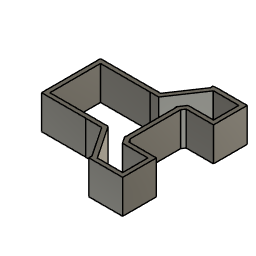
Duplex Sample Pad 1.5ScaleUp (Autodesk Fusion 360 design; units mm, degrees)
Autodesk Fusion 360 part; units mm, degrees
note: some values were not read from the file. Set by a fixed rule: which sketch regions a step uses.
sketch "Sketch1" plane through (0, 0, 0) normal (0, 0, 1) x (1, 0, 0)
  line L0 (5.0374, 3.1227) -> (6.2836, 3.1227)
  line L1 (6.2836, 3.1227) -> (6.2836, 5.3716)
  line L2 (6.2836, 5.3716) -> (4.024, 5.3716)
  line L3 (4.024, 5.3716) -> (4.024, 5.3478)
  line L4 (4.024, 5.3478) -> (2.0793, 2.4559)
  line L5 (2.0793, 2.4559) -> (1.3173, 2.4559)
  line L6 (1.3173, 2.4559) -> (1.3173, 2.4506)
  line L7 (1.3173, 2.4506) -> (-3.0986, 2.4506)
  line L8 (-3.0986, 2.4506) -> (-3.0986, -2.0499)
  line L9 (-3.0986, -2.0499) -> (0.9892, -2.0499)
  line L10 (0.9892, -2.0499) -> (0.9892, -2.0552)
  line L11 (0.9892, -2.0552) -> (2.0846, -2.0552)
  line L12 (2.0846, -2.0552) -> (4.0293, -4.9471)
  line L13 (4.0293, -4.9471) -> (4.0293, -4.9709)
  line L14 (4.0293, -4.9709) -> (6.2889, -4.9709)
  line L15 (6.2889, -4.9709) -> (6.2889, -2.722)
  line L16 (6.2889, -2.722) -> (5.0427, -2.722)
  line L17 (5.0427, -2.722) -> (4.0293, -2.722)
  line L18 (4.0293, -2.722) -> (3.5822, -2.0579)
  line L19 (3.5822, -2.0579) -> (3.6457, -2.0579)
  line L20 (3.6457, -2.0579) -> (3.6457, -2.0526)
  line L21 (3.6457, -2.0526) -> (3.6536, -2.0526)
  line L22 (3.6536, -2.0526) -> (3.6536, 2.448)
  line L23 (3.6536, 2.448) -> (3.6457, 2.448)
  line L24 (3.6457, 2.448) -> (3.6457, 2.4533)
  line L25 (3.6457, 2.4533) -> (3.5822, 2.4533)
  line L26 (3.5822, 2.4533) -> (4.0293, 3.1174)
  line L27 (4.0293, 3.1174) -> (5.0427, 3.1174)
  line L28 (5.0427, 3.1174) -> (5.0374, 3.1227)
  line L29 (4.2251, 2.7496) -> (6.6593, 2.7496)
  line L30 (6.6593, 2.7496) -> (6.6593, 5.75)
  line L31 (6.6593, 5.75) -> (4.024, 5.75)
  line L32 (4.024, 5.75) -> (3.6483, 5.7262)
  line L33 (3.6483, 5.7262) -> (3.6483, 5.4642)
  line L34 (3.6483, 5.4642) -> (1.8782, 2.8343)
  line L35 (1.8782, 2.8343) -> (1.3147, 2.8343)
  line L36 (1.3147, 2.8343) -> (0.9813, 2.829)
  line L37 (0.9813, 2.829) -> (-3.4743, 2.829)
  line L38 (-3.4743, 2.829) -> (-3.4743, -2.4204)
  line L39 (-3.4743, -2.4204) -> (0.4574, -2.4204)
  line L40 (0.4574, -2.4204) -> (0.4574, -2.4256)
  line L41 (0.4574, -2.4256) -> (1.8809, -2.4256)
  line L42 (1.8809, -2.4256) -> (3.651, -5.0556)
  line L43 (3.651, -5.0556) -> (3.651, -5.3387)
  line L44 (3.651, -5.3387) -> (6.6619, -5.3387)
  line L45 (6.6619, -5.3387) -> (6.6619, -2.3383)
  line L46 (6.6619, -2.3383) -> (4.2277, -2.3383)
  line L47 (4.2277, -2.3383) -> (4.0267, -2.0394)
  line L48 (4.0267, -2.0394) -> (4.0267, 2.4559)
  line L49 (4.0267, 2.4559) -> (4.2277, 2.7549)
  line L50 (4.2277, 2.7549) -> (4.2251, 2.7496)
  line L51 (3.6404, 2.4586) -> (3.6404, 2.4533)
  line L52 (3.6404, 2.4533) -> (3.6483, 2.4533)
  line L53 (3.6483, 2.4533) -> (3.6483, -2.0473)
  line L54 (3.6483, -2.0473) -> (3.6404, -2.0473)
  line L55 (3.6404, -2.0473) -> (3.6404, -2.0526)
  line L56 (3.6404, -2.0526) -> (3.5769, -2.0526)
  line L57 (3.5769, -2.0526) -> (4.024, -2.7167)
  line L58 (4.024, -2.7167) -> (5.0374, -2.7167)
  line L59 (5.0374, -2.7167) -> (6.2836, -2.7167)
  line L60 (6.2836, -2.7167) -> (6.2836, -4.9657)
  line L61 (6.2836, -4.9657) -> (4.024, -4.9657)
  line L62 (4.024, -4.9657) -> (4.024, -4.9418)
  line L63 (4.024, -4.9418) -> (2.0793, -2.0499)
  line L64 (2.0793, -2.0499) -> (0.9839, -2.0499)
  line L65 (0.9839, -2.0499) -> (0.9839, -2.0447)
  line L66 (0.9839, -2.0447) -> (-3.1039, -2.0447)
  line L67 (-3.1039, -2.0447) -> (-3.1039, 2.4559)
  line L68 (-3.1039, 2.4559) -> (1.312, 2.4559)
  line L69 (1.312, 2.4559) -> (1.312, 2.4612)
  line L70 (1.312, 2.4612) -> (2.074, 2.4612)
  line L71 (2.074, 2.4612) -> (4.0187, 5.3531)
  line L72 (4.0187, 5.3531) -> (4.0187, 5.3769)
  line L73 (4.0187, 5.3769) -> (6.2783, 5.3769)
  line L74 (6.2783, 5.3769) -> (6.2783, 3.1279)
  line L75 (6.2783, 3.1279) -> (5.0321, 3.1279)
  line L76 (5.0321, 3.1279) -> (4.0187, 3.1279)
  line L77 (4.0187, 3.1279) -> (3.5716, 2.4638)
extrude "Extrude1" add sketch "Sketch1" along normal blind 3
scale "Scale1" factor 1.5 about (2.0829, -2.0552, 3) bodies 1
